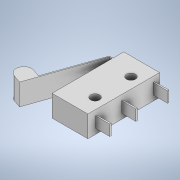
# Autodesk Inventor part: LimitSwitch
Saved by Autodesk Inventor 2022 (Build 260153000, 153)
## iProperties
Created: 2021-06-30
Part Number: LimitSwitch
Material: Generic
Document SubType Name: Modeling
Designer: BBL
Density: 1 g/cm^3
Appearance: Default
Author: BBL
Autodesk Inventor part; units mm, degrees
ref_plane "YZ Plane" through (0, 0, 0) normal (1, 0, 0) x (0, 1, 0)
ref_plane "XZ Plane" through (0, 0, 0) normal (0, 1, 0) x (-1, 0, 0)
ref_plane "XY Plane" through (0, 0, 0) normal (0, 0, 1) x (1, 0, 0)
sketch "Sketch1" plane through (0, 0, 0) normal (0, 1, 0) x (-1, 0, 0)
  line L0 (0, 0) -> (10, 0)
  line L1 (10, 0) -> (10, -20)
  line L2 (10, -20) -> (0, -20)
  line L3 (0, -20) -> (0, 0)
  circle A0 centre (3, -5) radius 1.25
  circle A1 centre (3, -15) radius 1.25
  dimension "d0" = 10
  dimension "d1" = 20
  dimension "d2" = 2.5
  dimension "d3" = 2.5
  dimension "d4" = 3
  dimension "d5" = 3
  dimension "d6" = 5
  dimension "d7" = 5
  constraints: 8 end point, 2 centre point, 2 parallel, 1 horizontal, 1 perpendicular
  measures "d0" distance of L1.end L2.end
  measures "d1" distance of L0.end L1.end
  measures "d2" diameter of A0
  measures "d3" diameter of A1
  measures "d4" distance from line of L3 A0.centre
  measures "d5" distance from line of L3 A1.centre
  measures "d6" distance from line of L0 A0.centre
  measures "d7" distance from line of L2 A1.centre
extrude "Extrusion1" add sketch "Sketch1" along normal blind 6
sketch "Sketch2" plane through (0, 6, 0) normal (0, 1, 0) x (1, 0, 0)
  line L0 (0, 20) -> (-10, 20) projected
  line L1 (-10, 20) -> (-10, 0) projected
  line L2 (-10, 0) -> (0, 0) projected
  line L3 (0, 0) -> (0, 20) projected
  circle A0 centre (-3, 15) radius 1.25 projected
  circle A1 centre (-3, 5) radius 1.25 projected
  circle A2 centre (-18.85, 1) radius 2.15
  line L4 (-10, 20) -> (-10, 0) projected
  line L5 (-10, 17) -> (-11, 17)
  line L6 (-11, 17) -> (-17.5269, -1.7376)
  line L7 (-16.1124, 2.3231) -> (-18.1428, 3.0303)
  line L8 (-19.5572, -1.0303) -> (-17.2436, -1.8363)
  line L9 (-17.2436, -1.8363) -> (-10.7868, 16.7)
  line L10 (-10.7868, 16.7) -> (-10, 16.7)
  dimension "d10" = 4.3
  dimension "d11" = 18.85
  dimension "d12" = 1
  dimension "d13" = 1
  dimension "d15" = 3
  dimension "d16" = 0.3
  dimension "d17" = 0.3
  constraints: 12 end point, 4 point on line, 3 tangent, 2 perpendicular, 2 point on circle, 1 centre point
  measures "d10" diameter of A2
  measures "d11" distance from line of L3 A2.centre
  measures "d12" distance from line of A2.centre L2
  measures "d13" distance of L5.start L5.end
  measures "d15" distance between parallel lines of L0 L5
  measures "d16" distance between parallel lines of L6 L9
  measures "d17" distance between parallel lines of L5 L10
extrude "Extrusion2" add sketch "Sketch2" against normal blind 6 contours L1 L10 L9 L8 L6 L5 | L6 A2 L7 | L6 L8 A2 | A2
sketch "Sketch3" plane through (0, 0, 0) normal (1, 0, 0) x (0, 0, -1)
  line L0 (2.1, 4.5) -> (2.5, 4.5)
  line L1 (2.5, 4.5) -> (2.5, 1.5)
  line L2 (2.5, 1.5) -> (2.1, 1.5)
  line L3 (2.1, 1.5) -> (2.1, 4.5)
  line L4 (0, 0) -> (20, 0) projected
  line L5 (20, 0) -> (20, 6) projected
  line L6 (0, 6) -> (20, 6) projected
  line L7 (0, 0) -> (0, 6) projected
  line L8 (9.4, 4.5) -> (9.8, 4.5)
  line L9 (9.8, 4.5) -> (9.8, 1.5)
  line L10 (9.8, 1.5) -> (9.4, 1.5)
  line L11 (9.4, 1.5) -> (9.4, 4.5)
  line L12 (18.2, 4.5) -> (18.6, 4.5)
  line L13 (18.6, 4.5) -> (18.6, 1.5)
  line L14 (18.6, 1.5) -> (18.2, 1.5)
  line L15 (18.2, 1.5) -> (18.2, 4.5)
  dimension "d20" = 3
  dimension "d21" = 3
  dimension "d22" = 3
  dimension "d23" = 0.4
  dimension "d24" = 0.4
  dimension "d25" = 0.4
  dimension "d26" = 1.5
  dimension "d27" = 1.5
  dimension "d28" = 2.5
  dimension "d29" = 7.7
  dimension "d31" = 16.5
  constraints: 24 end point, 6 parallel, 3 horizontal, 3 perpendicular, 1 point on line
  measures "d20" distance of L2.end L0.start
  measures "d21" distance of L10.end L8.start
  measures "d22" distance of L14.end L12.start
  measures "d23" distance of L0.start L0.end
  measures "d24" distance of L8.start L8.end
  measures "d25" distance of L12.start L12.end
  measures "d26" distance between parallel lines of L6 L0
  measures "d27" distance between parallel lines of L6 L8
  measures "d28" distance between parallel lines of L7 L1
  measures "d29" distance between parallel lines of L9 L3
  measures "d31" distance between parallel lines of L13 L3
extrude "Extrusion3" add sketch "Sketch3" along normal blind 4 contours L0 L1 L2 L3 | L8 L9 L10 L11 | L12 L13 L14 L15
equation "\"d21\" = d20"
equation "\"d22\" = d21"
equation "\"d24\" = d23"
equation "\"d25\" = d23"
equation "\"d27\" = d26"
body "Solid1"
